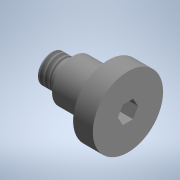
# Autodesk Inventor part: DBS4-5-5_AddProc
Saved by Autodesk Inventor 2020 (Build 240168000, 168)
## iProperties
Part Number: DBS4-5-5_AddProc
Material: 一般
Catalog Web Link: https://jp.misumi-ec.com/vona2/detail/110302403310/?HissuCode=DBS4-5-5
Description: 既製品
Vendor: MISUMI
Document SubType Name: Modeling
Designer: partserver
Manufacturer: MISUMI
Mass: 0.408326 g
Surface Area: 4.21132 cm^2
Volume: 0.408326 cm^3
Density: 1 g/cm^3
Appearance: PSOLRGB-175-175-175
Category: PARTsolutions
Company: MISUMI
PSOL_IDENT_0: {$CADENAS_DATA\23d-libs\misumi\metric\27_screws_nuts\dbb.prj},176 {VTYP=3D},{NB=DBS4-5-5},{LINA=DBS4
PSOL_IDENT_1: -5-5},{NN=DBB, DBM, DBS},{DATE=30.06.2021 13:09:28},{GEOMDATE=15.01.2020 08:58:15},{VERSION=},{LINEI
PSOL_IDENT_2: D=20},{WBVAR=MAT,ST,L,F},{WBNUMERIC=L,F}  {NB=DBS4-5-5},{LINA=DBS4-5-5},{KT=DUMMY},{PN=DBS4-5-5},{TY
PSOL_IDENT_3: PE=DB},{MAT=S},{ST=-},{STALG= '-','-'},{M=4},{L=5},{LALG=3,4,5,6,7,8,10},{F=5},{FALG=4,5,6,8},{E=2.8
PSOL_IDENT_4: },{DHH7=6},{A=10},{B=2.5},{LL=1.2},{HH1=2.5}
NB: DBS4-5-5
NN: DBB, DBM, DBS
NT: Stepped Screws - Low Head Selectable
NBSYN: $PN.
LINA: DBS4-5-5
CATALOG: Misumi
PN: DBS4-5-5
TYPE: DB
MAT: 303 Stainless Steel
ST: -
M: 4
L: 5
F: 5
E: 2.8
DHH7: 6
A: 10
B: 2.5
LL: 1.2
HH1: 2.5
SUPPLIER: MISUMI
ARTICLENO: DBS4-5-5
BOMINFO: DBS4-5-5
CREATOR: CADENAS GmbH
Title: DBS4-5-5
Author: Cadenas PARTsolutions
Autodesk Inventor part; units mm, degrees
ref_plane "YZ Plane" through (0, 0, 0) normal (1, 0, 0) x (0, 1, 0)
ref_plane "XZ Plane" through (0, 0, 0) normal (0, 1, 0) x (-1, 0, 0)
ref_plane "XY Plane" through (0, 0, 0) normal (0, 0, 1) x (1, 0, 0)
sketch "Sketch_1" plane through (0, 0, 0) normal (0, 0, 1) x (1, 0, 0)
  line L0 (5, 0) -> (-7.8, 0)
  line L1 (-7.8, 0) -> (-7.8, 5)
  line L2 (-7.8, 5) -> (-5, 5)
  line L3 (-5, 5) -> (-5, 3)
  line L4 (-5, 3) -> (0, 3)
  line L5 (0, 3) -> (0, 2)
  line L6 (0, 2) -> (4.5705, 2)
  line L7 (4.5705, 2) -> (5, 1.5705)
  line L8 (5, 1.5705) -> (5, 0)
  line L9 (5, 0) -> (-7.8, 0)
  constraints: 20 end point
revolve "Revolution1" add sketch "Sketch_1" angle 360 about axis through (5, 0, 0) along (1, 0, 0)
thread "Thread1" size "M4x0.7" class "6g" standard "ISO Metric profile" length 3.3705
sketch "Sketch_2" plane through (-7.8, 0, 0) normal (-1, 0, 0) x (0, 1, 0)
  line L0 (-1.4434, 0) -> (-0.7217, -1.25)
  line L1 (-0.7217, -1.25) -> (0.7217, -1.25)
  line L2 (0.7217, -1.25) -> (1.4434, 0)
  line L3 (1.4434, 0) -> (0.7217, 1.25)
  line L4 (0.7217, 1.25) -> (-0.7217, 1.25)
  line L5 (-0.7217, 1.25) -> (-1.4434, 0)
  constraints: 12 end point
extrude "Extrusion1" cut sketch "Sketch_2" against normal blind 2.5
sketch "Sketch_3" plane through (0, 0, 0) normal (0, 0, 1) x (1, 0, 0)
  line L0 (-4.5783, 0) -> (-5.3, 0)
  line L1 (-5.3, 0) -> (-5.3, 1.25)
  line L2 (-5.3, 1.25) -> (-4.5783, 0)
  line L3 (-4.5783, 0) -> (-5.3, 0)
  constraints: 8 end point
revolve "Revolution2" cut sketch "Sketch_3" angle 360 about axis through (-4.5783, 0, 0) along (1, 0, 0)
sketch "スケッチ4" plane through (5, 0, 0) normal (1, 0, 0) x (0, 0, -1)
  circle A0 centre (0, 0) radius 5
  constraints: 1 centre point, 1 coincident
extrude "押し出し2" cut sketch "スケッチ4" against normal blind 2
body "Solid1"
